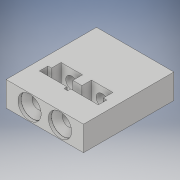
# Autodesk Inventor part: base1
Saved by Autodesk Inventor 2019 (Build 230136000, 136)
## iProperties
Created: 2019-10-15
Part Number: base1
Material: Générique
Document SubType Name: Modeling
Designer: dubicube
Density: 1 g/cm^3
Appearance: Par défaut
Author: dubicube
Autodesk Inventor part; units mm, degrees
ref_plane "YZ Plane" through (0, 0, 0) normal (1, 0, 0) x (0, 1, 0)
ref_plane "XZ Plane" through (0, 0, 0) normal (0, 1, 0) x (-1, 0, 0)
ref_plane "XY Plane" through (0, 0, 0) normal (0, 0, 1) x (1, 0, 0)
sketch "Esquisse1" plane through (0, 0, 0) normal (0, 1, 0) x (-1, 0, 0)
  line L0 (12.8426, 45) -> (-12.8426, 45)
  line L1 (-12.8426, 45) -> (-12.8426, 75)
  line L2 (-12.8426, 75) -> (12.8426, 75)
  line L3 (12.8426, 75) -> (12.8426, 45)
  line L4 (9.75, 67) -> (-9.75, 67)
  line L5 (-9.75, 67) -> (-9.75, 64.2)
  line L6 (-9.75, 64.2) -> (9.75, 64.2)
  line L7 (9.75, 64.2) -> (9.75, 67)
  line L8 (0, -15) -> (0, 90) projected
  point P0 (0, 0)
  point P1 (0, 64.2)
  point P2 (0, 45)
  dimension "d0" = 75
  dimension "d1" = 19.5
  dimension "d2" = 2.8
  dimension "d3" = 8
  dimension "d45" = 30
  dimension "d46" = 25.6852
  constraints: 16 end point, 4 parallel, 2 horizontal, 2 midpoint, 2 perpendicular, 2 point on line
  measures "d0" distance from line of L2 point (0, 0)
  measures "d1" distance of L5.end L6.end
  measures "d2" distance of L4.end L5.end
  measures "d3" distance between parallel lines of L2 L4
  measures "d45" distance of L2.end L0.start
  measures "d46" distance of L0.start L0.end
extrude "Extrusion1" add sketch "Esquisse1" along normal mid plane 8.2 contours L0 L8 L6 L7 L4 L2 L3 | L0 L1 L2 L8 L4 L5 L6
sketch "Esquisse2" plane through (-12.8426, -4.1, 75) normal (0, 0, 1) x (1, 0, 0)
  circle A0 centre (17.8926, 4.1) radius 3.85
  circle A1 centre (7.7926, 4.1) radius 3.85
  line L0 (17.8926, 4.1) -> (7.7926, 4.1) construction
  line L1 (12.8426, -1.64) -> (12.8426, 9.84) construction
  point P0 (12.8426, 4.1)
  dimension "d6" = 7.7
  dimension "d7" = 10.1
  constraints: 2 centre point, 2 end point, 1 equal radius, 1 horizontal, 1 midpoint
  measures "d6" diameter of A1
  measures "d7" distance of L0.end L0.start
extrude "Extrusion2" cut sketch "Esquisse2" against normal blind 1
sketch "Esquisse3" plane through (-12.8426, -4.1, 74) normal (0, 0, 1) x (1, 0, 0)
  circle A0 centre (7.7926, 4.1) radius 3.85 projected
  circle A1 centre (7.7926, 4.1) radius 2
  circle A2 centre (17.8926, 4.1) radius 3.85 projected
  circle A3 centre (17.8926, 4.1) radius 2
  point P0 (12.8426, 4.1)
  point P1 (9.3965, 7)
  point P2 (9.3965, 0)
  point P3 (16.2887, 0)
  point P4 (16.2887, 7)
  dimension "d10" = 4
  dimension "d11" = 4
  constraints: 2 centre point, 2 coincident, 2 other
  measures "d10" diameter of A1
  measures "d11" diameter of A3
extrude "Extrusion3" cut sketch "Esquisse3" against normal blind 20 contours A1 | A3
chamfer "Chanfrein1" distance 1.8 angle 45 2 edges at (-7.05, 0, 74) (3.05, 0, 74)
sketch "Esquisse5" plane through (0, 4.1, 0) normal (0, 1, 0) x (1, 0, 0)
  line L0 (-9.75, -64.2) -> (9.75, -64.2) projected
  line L1 (-8.6, -64.2) -> (-1.5, -64.2)
  line L2 (-1.5, -64.2) -> (-1.5, -61)
  line L3 (-1.5, -61) -> (-8.6, -61)
  line L4 (-8.6, -61) -> (-8.6, -64.2)
  line L5 (1.5, -64.2) -> (8.6, -64.2)
  line L6 (8.6, -64.2) -> (8.6, -61)
  line L7 (8.6, -61) -> (1.5, -61)
  line L8 (1.5, -61) -> (1.5, -64.2)
  line L9 (5.05, 15) -> (5.05, -90) projected
  line L10 (-5.05, 15) -> (-5.05, -90) projected
  line L11 (9.75, -67) -> (-9.75, -67) projected
  line L12 (-0.6, -67) -> (0.6, -67)
  line L13 (0.6, -67) -> (0.6, -68)
  line L14 (0.6, -68) -> (-0.6, -68)
  line L15 (-0.6, -68) -> (-0.6, -67)
  point P0 (0, 0)
  point P1 (5.05, -64.2)
  point P2 (-5.05, -64.2)
  point P3 (0, -67)
  dimension "d17" = 7.1
  dimension "d18" = 3.2
  dimension "d19" = 3.2
  dimension "d22" = 1.2
  dimension "d24" = 1
  constraints: 24 end point, 6 parallel, 5 point on line, 4 midpoint, 3 horizontal, 3 perpendicular, 1 collinear
  measures "d17" distance of L2.end L3.end
  measures "d18" distance of L3.end L1.start
  measures "d19" distance of L7.end L5.start
  measures "d22" distance of L13.end L14.end
  measures "d24" distance of L12.end L13.end
extrude "Extrusion4" cut sketch "Esquisse5" against normal blind 20 contours L0 L10 L3 L2 | L8 L7 L9 L0 | L0 L4 L3 L10 | L9 L7 L6 L0 | L11 L13 L14 L15
